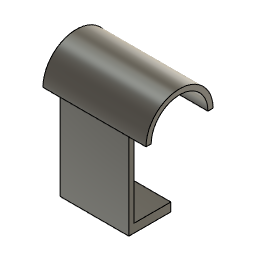
CameraHolder v1 (Autodesk Fusion 360 design; units mm, degrees)
Autodesk Fusion 360 part; units mm, degrees
sketch "Sketch2" plane through (0, 0, 0) normal (0, 0, 1) x (1, 0, 0)
  line L0 (0, 0) -> (40, 0)
  line L1 (40, 0) -> (40, 24.4086)
  line L2 (40, 24.4086) -> (0, 24.4086)
  line L3 (0, 24.4086) -> (0, 0)
  constraint horizontal L0
  constraint vertical L1
  constraint horizontal L2
  constraint vertical L3
  constraint coincident L0.start L3.end
extrude "Extrude1" add sketch "Sketch2" along normal blind 5
sketch "Sketch3" plane through (0, 0, 0) normal (0, -1, 0) x (1, 0, 0)
  line L0 (0, 0) -> (40, 0)
  line L1 (40, 0) -> (40, 5)
  line L2 (40, 5) -> (0, 5)
  line L3 (0, 5) -> (0, 0)
  line L4 (0, 0) -> (40, 0)
  line L5 (40, 0) -> (40, 50)
  line L6 (40, 50) -> (0, 50)
  line L7 (0, 50) -> (0, 0)
  constraint horizontal L4
  constraint vertical L5
  constraint horizontal L6
  constraint vertical L7
  constraint coincident L0.start L3.end
extrude "Extrude2" add sketch "Sketch3" against normal blind 3 contours L2 L5 L6 L7
sketch "Sketch4" plane through (40, 0, 0) normal (1, 0, 0) x (0, 1, 0)
  line L0 (0, 0) -> (24.4086, 0)
  line L1 (24.4086, 0) -> (24.4086, 5)
  line L2 (24.4086, 5) -> (3, 5)
  line L3 (3, 5) -> (3, 50)
  line L4 (3, 50) -> (0, 50)
  line L5 (0, 50) -> (0, 0)
  line L6 (19.5, 40) -> (19.5, 70) construction
  arc A0 (36, 50) -> (3, 50) centre (19.5, 50) ccw
  arc A1 (39, 50) -> (0, 50) centre (19.5, 50) ccw
  line L7 (36, 50) -> (39, 50)
  line L8 (36, 50) -> (39, 50)
  line L9 (0, 50) -> (3, 50)
  dimension "d7" = 16.5
  dimension "d8" = 3
  constraint perpendicular L4 L6
  constraint coincident L3.end L4.start
  constraint coincident L6 A0.centre
  constraint perpendicular L3 L9
  measures "d7" distance of L3 L6
extrude "Extrude3" add sketch "Sketch4" along normal blind 10 and the other way blind 50 contours L4 A0 A1 L7 L8 L9
equation "d7 = ( 33 / 2 ) * 1 mm"
